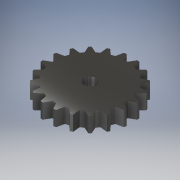
# Autodesk Inventor part: Part11
Saved by Autodesk Inventor 2019 (Build 230136000, 136)
## iProperties
Created: 2022-01-28
Part Number: Part11
Material: Generic
Document SubType Name: Modeling
Designer: Sepehr
Density: 1 g/cm^3
Appearance: Default
Author: Sepehr
Autodesk Inventor part; units mm, degrees
ref_plane "YZ Plane" through (0, 0, 0) normal (1, 0, 0) x (0, 1, 0)
ref_plane "XZ Plane" through (0, 0, 0) normal (0, 1, 0) x (-1, 0, 0)
ref_plane "XY Plane" through (0, 0, 0) normal (0, 0, 1) x (1, 0, 0)
sketch "Sketch1" plane through (0, 0, 0) normal (0, 1, 0) x (-1, 0, 0)
  circle A0 centre (0, 0) radius 3550
  line L0 (0, 0) -> (0, -150)
  line L1 (0, 150) -> (0, -150)
  line L2 (4243.0122, 0) -> (4511.7157, 0) construction
  line L3 (0, 0) -> (0, 150)
  arc A1 (2996.2477, -150) -> (2996.2477, 150) centre (0, 0) ccw
  line L4 (2996.2477, -150) -> (3520.9843, -452.9568)
  line L5 (2996.2477, 150) -> (3520.9843, 452.9568)
  point P0 (3536.4628, -309.7269)
  point P1 (3536.4628, 309.7269)
  dimension "d1" = 150
  dimension "d20" = 150
  constraints: 12 end point, 6 point on circle, 2 centre point, 1 coincident, 1 collinear, 1 horizontal, 1 point on line, 1 vertical
  measures "d1" distance of L0.start L0.end
  measures "d20" distance of L0.start L1.start
ref_plane "Work Plane1" through (0, 625, 0) normal (0, 1, 0) x (1, 0, 0)
extrude "Extrusion4" add sketch "Sketch1" along normal blind 1250
extrude "Extrusion5" cut sketch "Sketch1" along normal blind 1250 contours A0 L4 A1 L5 picked at (3349.0246, 326.912)
pattern_circular "Circular Pattern2" count 20 over 360 about axis through (0, -10, 0) along (0, 1, 0) of "Extrusion5"
sketch "Sketch3" plane through (0, 1250, 0) normal (0, 1, 0) x (1, 0, 0)
  arc A0 (484.1229, 125) -> (484.1229, -125) centre (0, 0) ccw
  line L0 (484.1229, -125) -> (600, -125)
  line L1 (600, -125) -> (600, 125)
  line L2 (600, 125) -> (484.1229, 125)
  constraints: 6 end point, 2 perpendicular, 2 point on circle, 1 centre point
extrude "Extrusion7" cut sketch "Sketch3" against normal blind 1250
body "Solid1"
